Autodesk Fusion 360 part; units mm, degrees
(part 2 of 2)
sketch "Skizze4" plane through (0, 0, 0) normal (0, 1, 0) x (1, 0, 0)
  line L0 (145, 5) -> (150, 5)
  line L1 (150, 5) -> (150, 0)
  line L2 (150, 0) -> (230, 0)
  line L3 (230, 0) -> (230, 5)
  line L4 (230, 5) -> (235, 5)
  line L5 (235, 5) -> (235, 100)
  line L6 (235, 100) -> (145, 100)
  line L7 (145, 100) -> (145, 5)
  line L8 (125, 35) -> (125.0002, 27.0709)
  line L9 (117.9289, 20) -> (137.9289, 0)
  line L10 (145, 0) -> (148.5355, 3.5355) construction
  line L11 (152.0711, 0) -> (172.0709, 19.9998)
  line L12 (165, 35) -> (165, 27.0711)
  line L13 (145, 7.0711) -> (125.0002, 27.0709)
  line L14 (148.5355, -3.5355) -> (180.4271, 28.356) construction
  line L15 (141.4645, 3.5355) -> (172.9289, 35) construction
  line L16 (180, 20) -> (172.0709, 19.9998)
  line L17 (145, 0) -> (141.4645, 3.5355) construction
  line L18 (145, 0) -> (148.5355, -3.5355) construction
  line L19 (141.4645, -3.5355) -> (110, 27.9289) construction
  line L20 (145, -7.0711) -> (164.9998, -27.0709)
  line L21 (141.4645, -3.5355) -> (172.9289, -35) construction
  line L22 (172.0711, -20) -> (152.0711, 0)
  line L23 (110, 35) -> (180, 35) construction
  line L24 (148.5355, -3.5355) -> (117.0711, -35) construction
  line L25 (180, -35) -> (180, -20)
  line L26 (117.9291, -19.9998) -> (110, -19.9998)
  line L27 (180, -35) -> (110, -35) construction
  line L28 (150, 0) -> (150, -5)
  line L29 (180, 20) -> (180, 35)
  line L30 (145, 0) -> (141.4645, -3.5355) construction
  line L31 (180, 35) -> (165, 35)
  line L32 (165, 27.0711) -> (145, 7.0711)
  line L33 (180, 35) -> (110, -35) construction
  line L34 (150, -5) -> (145, -5)
  line L35 (172.0711, -20) -> (180, -20)
  line L36 (164.9998, -35) -> (164.9998, -27.0709)
  line L37 (110, 35) -> (180, -35) construction
  line L38 (110, -35) -> (125, -35)
  line L39 (110, -35) -> (110, 35) construction
  line L40 (164.9998, -35) -> (180, -35)
  line L41 (125, -35) -> (125, -27.0711)
  line L42 (110, -19.9998) -> (110, -35)
  line L43 (110, 35) -> (110, 20)
  line L44 (125, 35) -> (110, 35)
  line L45 (141.4645, 3.5355) -> (110, -27.9289) construction
  line L46 (110, 20) -> (117.9289, 20)
  line L47 (148.5355, 3.5355) -> (180, -27.9289) construction
  line L48 (137.9289, 0) -> (117.9291, -19.9998)
  line L49 (148.5355, 3.5355) -> (117.0711, 35) construction
  line L50 (180, 35) -> (180, -35) construction
  line L51 (125, -27.0711) -> (145, -7.0711)
  line L52 (215, 35) -> (215.0002, 27.0709)
  line L53 (207.9289, 20) -> (227.9289, 0)
  line L54 (235, 0) -> (238.5355, 3.5355) construction
  line L55 (242.0711, 0) -> (262.0709, 19.9998)
  line L56 (255, 35) -> (255, 27.0711)
  line L57 (235, 7.0711) -> (215.0002, 27.0709)
  line L58 (238.5355, -3.5355) -> (270.4271, 28.356) construction
  line L59 (231.4645, 3.5355) -> (262.9289, 35) construction
  line L60 (270, 20) -> (262.0709, 19.9998)
  line L61 (235, 0) -> (231.4645, 3.5355) construction
  line L62 (235, 0) -> (238.5355, -3.5355) construction
  line L63 (231.4645, -3.5355) -> (200, 27.9289) construction
  line L64 (235, -7.0711) -> (254.9998, -27.0709)
  line L65 (231.4645, -3.5355) -> (262.9289, -35) construction
  line L66 (262.0711, -20) -> (242.0711, 0)
  line L67 (200, 35) -> (270, 35) construction
  line L68 (238.5355, -3.5355) -> (207.0711, -35) construction
  line L69 (270, -35) -> (270, -20)
  line L70 (207.9291, -19.9998) -> (200, -19.9998)
  line L71 (270, -35) -> (200, -35) construction
  line L72 (240, 0) -> (240, -5)
  line L73 (270, 20) -> (270, 35)
  line L74 (235, 0) -> (231.4645, -3.5355) construction
  line L75 (270, 35) -> (255, 35)
  line L76 (255, 27.0711) -> (235, 7.0711)
  line L77 (270, 35) -> (200, -35) construction
  line L78 (240, -5) -> (235, -5)
  line L79 (262.0711, -20) -> (270, -20)
  line L80 (254.9998, -35) -> (254.9998, -27.0709)
  line L81 (200, 35) -> (270, -35) construction
  line L82 (200, -35) -> (215, -35)
  line L83 (200, -35) -> (200, 35) construction
  line L84 (254.9998, -35) -> (270, -35)
  line L85 (215, -35) -> (215, -27.0711)
  line L86 (200, -19.9998) -> (200, -35)
  line L87 (200, 35) -> (200, 20)
  line L88 (215, 35) -> (200, 35)
  line L89 (231.4645, 3.5355) -> (200, -27.9289) construction
  line L90 (200, 20) -> (207.9289, 20)
  line L91 (238.5355, 3.5355) -> (270, -27.9289) construction
  line L92 (227.9289, 0) -> (207.9291, -19.9998)
  line L93 (238.5355, 3.5355) -> (207.0711, 35) construction
  line L94 (270, 35) -> (270, -35) construction
  line L95 (215, -27.0711) -> (235, -7.0711)
  line L96 (145, 85) -> (150, 85)
  line L97 (150, 85) -> (150, 95)
  line L98 (150, 95) -> (145, 95)
  line L99 (145, 95) -> (145, 85)
  line L100 (235, 95) -> (230, 95)
  line L101 (230, 95) -> (230, 85)
  line L102 (230, 85) -> (235, 85)
  line L103 (235, 85) -> (235, 95)
  dimension "d109" = 5
  dimension "d110" = 5
  dimension "d111" = 80
  dimension "d112" = 5
  dimension "d113" = 5
  dimension "d115" = 95
  dimension "d116" = 90
  dimension "d117" = 5
  dimension "d118" = 5
  dimension "d119" = 70
  dimension "d120" = 70
  dimension "d121" = 5
  dimension "d122" = 5
  dimension "d123" = 5
  dimension "d124" = 5
  dimension "d125" = 15
  dimension "d126" = 28.284
  dimension "d127" = 28.284
  dimension "d128" = 28.284
  dimension "d129" = 28.284
  dimension "d130" = 5
  dimension "d131" = 5
  dimension "d132" = 70
  dimension "d133" = 70
  dimension "d134" = 5
  dimension "d135" = 5
  dimension "d136" = 5
  dimension "d137" = 5
  dimension "d138" = 15
  dimension "d139" = 28.284
  dimension "d140" = 28.284
  dimension "d141" = 28.284
  dimension "d142" = 28.284
  dimension "d143" = 5
  dimension "d144" = 10
  dimension "d145" = 5
  dimension "d146" = 10
  constraint horizontal L0
  constraint perpendicular L0 L1
  constraint perpendicular L1 L2
  constraint perpendicular L2 L3
  constraint perpendicular L3 L4
  constraint perpendicular L4 L5
  constraint perpendicular L5 L6
  constraint horizontal L23
  constraint vertical L50
  constraint horizontal L27
  constraint vertical L39
  constraint midpoint L10.start L33
  constraint perpendicular L17 L33
  constraint coincident L15.end L23
  constraint perpendicular L15 L37
  constraint coincident L45.end L39
  constraint perpendicular L17 L45
  constraint perpendicular L18 L33
  constraint coincident L24.end L27
  constraint perpendicular L18 L24
  constraint perpendicular L14 L18
  constraint coincident L10.end L33
  constraint coincident L47.end L50
  constraint perpendicular L10 L47
  constraint coincident L49.end L23
  constraint perpendicular L10 L49
  constraint perpendicular L17 L30
  constraint coincident L21.end L27
  constraint perpendicular L21 L33
  constraint coincident L19.end L39
  constraint perpendicular L19 L33
  constraint perpendicular L23 L43
  constraint coincident L9.start L19
  constraint perpendicular L39 L46
  constraint coincident L9.end L19
  constraint coincident L9.end L45
  constraint coincident L26.start L45
  constraint coincident L26.end L39
  constraint perpendicular L26 L39
  constraint coincident L38.end L27
  constraint perpendicular L38 L42
  constraint coincident L41.end L24
  constraint perpendicular L27 L41
  constraint coincident L20.start L21
  constraint coincident L20.start L24
  constraint perpendicular L21 L51
  constraint perpendicular L20 L51
  constraint coincident L36.start L27
  constraint perpendicular L27 L36
  constraint coincident L25.end L50
  constraint perpendicular L25 L40
  constraint coincident L22.start L47
  constraint perpendicular L25 L35
  constraint coincident L11.start L47
  constraint coincident L11.start L14
  constraint perpendicular L14 L22
  constraint perpendicular L11 L47
  constraint coincident L16.start L50
  constraint coincident L12.start L23
  constraint perpendicular L31 L50
  constraint coincident L12.end L15
  constraint perpendicular L12 L23
  constraint coincident L13.start L49
  constraint coincident L13.start L15
  constraint perpendicular L32 L49
  constraint perpendicular L13 L32
  constraint coincident L8.start L23
  constraint horizontal L67
  constraint vertical L94
  constraint horizontal L71
  constraint vertical L83
  constraint midpoint L54.start L77
  constraint perpendicular L61 L77
  constraint coincident L59.end L67
  constraint perpendicular L59 L81
  constraint coincident L89.end L83
  constraint perpendicular L61 L89
  constraint perpendicular L62 L77
  constraint coincident L68.end L71
  constraint perpendicular L62 L68
  constraint perpendicular L58 L62
  constraint coincident L54.end L77
  constraint coincident L91.end L94
  constraint perpendicular L54 L91
  constraint coincident L93.end L67
  constraint perpendicular L54 L93
  constraint perpendicular L61 L74
  constraint coincident L65.end L71
  constraint perpendicular L65 L77
  constraint coincident L63.end L83
  constraint perpendicular L63 L77
  constraint perpendicular L67 L87
  constraint coincident L53.start L63
  constraint perpendicular L83 L90
  constraint coincident L53.end L63
  constraint coincident L53.end L89
  constraint coincident L70.start L89
  constraint coincident L70.end L83
  constraint perpendicular L70 L83
  constraint coincident L82.end L71
  constraint perpendicular L82 L86
  constraint coincident L85.end L68
  constraint perpendicular L71 L85
  constraint coincident L64.start L65
  constraint coincident L64.start L68
  constraint perpendicular L65 L95
  constraint perpendicular L64 L95
  constraint coincident L80.start L71
  constraint perpendicular L71 L80
  constraint coincident L69.end L94
  constraint perpendicular L69 L84
  constraint coincident L66.start L91
  constraint perpendicular L69 L79
  constraint coincident L55.start L91
  constraint coincident L55.start L58
  constraint perpendicular L58 L66
  constraint perpendicular L55 L91
  constraint coincident L60.start L94
  constraint coincident L56.start L67
  constraint perpendicular L75 L94
  constraint coincident L56.end L59
  constraint perpendicular L56 L67
  constraint coincident L57.start L93
  constraint coincident L57.start L59
  constraint perpendicular L76 L93
  constraint perpendicular L57 L76
  constraint coincident L52.start L67
  constraint horizontal L96
  constraint vertical L97
  constraint horizontal L98
  constraint vertical L99
  constraint coincident L7 L96.start
  constraint horizontal L100
  constraint vertical L101
  constraint horizontal L102
  constraint vertical L103
  constraint coincident L5 L100.start
  measures "d109" distance of L0.start L0.end
  measures "d110" distance of L0.end L1.end
  measures "d111" distance of L1.end L2.end
  measures "d112" distance of L2.end L3.end
  measures "d113" distance of L3.end L4.end
  measures "d115" distance of L4.end L5.end
  measures "d116" distance of L5.end L6.end
  measures "d117" distance of L28.end L1.end
  measures "d118" distance of L34.end L28.end
  measures "d119" distance of L23.end L23.start
  measures "d120" distance of L27.end L23.start
  measures "d121" distance of L10.start L15.start
  measures "d122" distance of L10.start L14.start
  measures "d123" distance of L10.end L10.start
  measures "d124" distance of L10.start L19.start
  measures "d125" distance of L23.start L43.end
  measures "d126" distance of L26.start L9.end
  measures "d127" distance of L20.start L20.end
  measures "d128" distance of L11.start L11.end
  measures "d129" distance of L8.end L13.start
  measures "d130" distance of L72.end L72.start
  measures "d131" distance of L78.end L72.end
  measures "d132" distance of L67.end L67.start
  measures "d133" distance of L71.end L67.start
  measures "d134" distance of L54.start L59.start
  measures "d135" distance of L54.start L58.start
  measures "d136" distance of L54.end L54.start
  measures "d137" distance of L54.start L63.start
  measures "d138" distance of L67.start L87.end
  measures "d139" distance of L70.start L53.end
  measures "d140" distance of L64.start L64.end
  measures "d141" distance of L55.start L55.end
  measures "d142" distance of L52.end L57.start
  measures "d143" distance of L96.start L96.end
  measures "d144" distance of L96.start L98.end
  measures "d145" distance of L100.start L100.end
  measures "d146" distance of L100.start L102.end
extrude "Extrusion4" add sketch "Skizze4" along normal blind 10 separate body contours L2 L5 L6 L7 L11 L12 L16 L29 L31 L32 L52 L53 L57 L87 L88 L90 L96 L97 L98 L100 L101 L102 makes body 4
sketch "Skizze5" plane through (0, 0, 0) normal (0, 1, 0) x (1, 0, 0)
  line L0 (145, 5) -> (150, 5)
  line L1 (150, 5) -> (150, 0)
  line L2 (150, 0) -> (230, 0)
  line L3 (230, 0) -> (230, 5)
  line L4 (230, 5) -> (235, 5)
  line L5 (235, 5) -> (235, 45)
  line L6 (235, 45) -> (145, 45)
  line L7 (145, 45) -> (145, 5)
  constraint horizontal L0
  constraint perpendicular L0 L1
  constraint perpendicular L1 L2
  constraint perpendicular L2 L3
  constraint perpendicular L3 L4
  constraint perpendicular L2 L5
  constraint perpendicular L5 L6
  constraint perpendicular L0 L7
extrude "Extrusion5" add sketch "Skizze5" along normal blind 5 bodies 4
sketch "Skizze6" plane through (0, 0, 0) normal (0, 1, 0) x (1, 0, 0)
  line L0 (320, 5) -> (325, 5)
  line L1 (325, 5) -> (325, 0)
  line L2 (325, 0) -> (420, 0)
  line L3 (420, 0) -> (420, 100)
  line L4 (420, 100) -> (320, 100)
  line L5 (320, 100) -> (320, 5)
  line L6 (300, 35) -> (300.0002, 27.0709)
  line L7 (292.9289, 20) -> (312.9289, 0)
  line L8 (320, 0) -> (323.5355, 3.5355) construction
  line L9 (327.0711, 0) -> (347.0709, 19.9998)
  line L10 (340, 35) -> (340, 27.0711)
  line L11 (320, 7.0711) -> (300.0002, 27.0709)
  line L12 (323.5355, -3.5355) -> (355.4271, 28.356) construction
  line L13 (316.4645, 3.5355) -> (347.9289, 35) construction
  line L14 (355, 20) -> (347.0709, 19.9998)
  line L15 (320, 0) -> (316.4645, 3.5355) construction
  line L16 (320, 0) -> (323.5355, -3.5355) construction
  line L17 (316.4645, -3.5355) -> (285, 27.9289) construction
  line L18 (320, -7.0711) -> (339.9998, -27.0709)
  line L19 (316.4645, -3.5355) -> (347.9289, -35) construction
  line L20 (347.0711, -20) -> (327.0711, 0)
  line L21 (285, 35) -> (355, 35) construction
  line L22 (323.5355, -3.5355) -> (292.0711, -35) construction
  line L23 (355, -35) -> (355, -20)
  line L24 (292.9291, -19.9998) -> (285, -19.9998)
  line L25 (355, -35) -> (285, -35) construction
  line L26 (325, 0) -> (325, -5)
  line L27 (355, 20) -> (355, 35)
  line L28 (320, 0) -> (316.4645, -3.5355) construction
  line L29 (355, 35) -> (340, 35)
  line L30 (340, 27.0711) -> (320, 7.0711)
  line L31 (355, 35) -> (285, -35) construction
  line L32 (325, -5) -> (320, -5)
  line L33 (347.0711, -20) -> (355, -20)
  line L34 (339.9998, -35) -> (339.9998, -27.0709)
  line L35 (285, 35) -> (355, -35) construction
  line L36 (285, -35) -> (300, -35)
  line L37 (285, -35) -> (285, 35) construction
  line L38 (339.9998, -35) -> (355, -35)
  line L39 (300, -35) -> (300, -27.0711)
  line L40 (285, -19.9998) -> (285, -35)
  line L41 (285, 35) -> (285, 20)
  line L42 (300, 35) -> (285, 35)
  line L43 (316.4645, 3.5355) -> (285, -27.9289) construction
  line L44 (285, 20) -> (292.9289, 20)
  line L45 (323.5355, 3.5355) -> (355, -27.9289) construction
  line L46 (312.9289, 0) -> (292.9291, -19.9998)
  line L47 (323.5355, 3.5355) -> (292.0711, 35) construction
  line L48 (355, 35) -> (355, -35) construction
  line L49 (300, -27.0711) -> (320, -7.0711)
  line L50 (320, 95) -> (325, 95)
  line L51 (325, 95) -> (325, 85)
  line L52 (325, 85) -> (320, 85)
  line L53 (320, 85) -> (320, 95)
  line L54 (415, 0) -> (405, 0)
  line L55 (405, 0) -> (405, 5)
  line L56 (405, 5) -> (415, 5)
  line L57 (415, 5) -> (415, 0)
  line L58 (415, 95) -> (405, 95)
  line L59 (405, 95) -> (405, 85)
  line L60 (405, 85) -> (415, 85)
  line L61 (415, 85) -> (415, 95)
  dimension "d151" = 95
  dimension "d152" = 100
  dimension "d153" = 100
  dimension "d154" = 5
  dimension "d155" = 5
  dimension "d156" = 70
  dimension "d157" = 70
  dimension "d158" = 5
  dimension "d159" = 5
  dimension "d160" = 5
  dimension "d161" = 5
  dimension "d162" = 15
  dimension "d163" = 28.284
  dimension "d164" = 28.284
  dimension "d165" = 28.284
  dimension "d166" = 28.284
  dimension "d167" = 5
  dimension "d168" = 10
  dimension "d169" = 10
  dimension "d170" = 5
  dimension "d171" = 10
  dimension "d172" = 10
  constraint horizontal L0
  constraint perpendicular L0 L1
  constraint perpendicular L1 L2
  constraint perpendicular L0 L3
  constraint perpendicular L3 L4
  constraint horizontal L21
  constraint vertical L48
  constraint horizontal L25
  constraint vertical L37
  constraint midpoint L8.start L31
  constraint perpendicular L15 L31
  constraint coincident L13.end L21
  constraint perpendicular L13 L35
  constraint coincident L43.end L37
  constraint perpendicular L15 L43
  constraint perpendicular L16 L31
  constraint coincident L22.end L25
  constraint perpendicular L16 L22
  constraint perpendicular L12 L16
  constraint coincident L8.end L31
  constraint coincident L45.end L48
  constraint perpendicular L8 L45
  constraint coincident L47.end L21
  constraint perpendicular L8 L47
  constraint perpendicular L15 L28
  constraint coincident L19.end L25
  constraint perpendicular L19 L31
  constraint coincident L17.end L37
  constraint perpendicular L17 L31
  constraint perpendicular L21 L41
  constraint coincident L7.start L17
  constraint perpendicular L37 L44
  constraint coincident L7.end L17
  constraint coincident L7.end L43
  constraint coincident L24.start L43
  constraint coincident L24.end L37
  constraint perpendicular L24 L37
  constraint coincident L36.end L25
  constraint perpendicular L36 L40
  constraint coincident L39.end L22
  constraint perpendicular L25 L39
  constraint coincident L18.start L19
  constraint coincident L18.start L22
  constraint perpendicular L19 L49
  constraint perpendicular L18 L49
  constraint coincident L34.start L25
  constraint perpendicular L25 L34
  constraint coincident L23.end L48
  constraint perpendicular L23 L38
  constraint coincident L20.start L45
  constraint perpendicular L23 L33
  constraint coincident L9.start L45
  constraint coincident L9.start L12
  constraint perpendicular L12 L20
  constraint perpendicular L9 L45
  constraint coincident L14.start L48
  constraint coincident L10.start L21
  constraint perpendicular L29 L48
  constraint coincident L10.end L13
  constraint perpendicular L10 L21
  constraint coincident L11.start L47
  constraint coincident L11.start L13
  constraint perpendicular L30 L47
  constraint perpendicular L11 L30
  constraint coincident L6.start L21
  constraint horizontal L50
  constraint vertical L51
  constraint horizontal L52
  constraint vertical L53
  constraint coincident L5 L50.start
  constraint horizontal L54
  constraint vertical L55
  constraint horizontal L56
  constraint vertical L57
  constraint coincident L2 L54.start
  constraint horizontal L58
  constraint vertical L59
  constraint horizontal L60
  constraint vertical L61
  measures "d151" distance of L1.end L2.end
  measures "d152" distance of L2.end L3.end
  measures "d153" distance of L3.end L4.end
  measures "d154" distance of L26.end L1.end
  measures "d155" distance of L32.end L26.end
  measures "d156" distance of L21.end L21.start
  measures "d157" distance of L25.end L21.start
  measures "d158" distance of L8.start L13.start
  measures "d159" distance of L8.start L12.start
  measures "d160" distance of L8.end L8.start
  measures "d161" distance of L8.start L17.start
  measures "d162" distance of L21.start L41.end
  measures "d163" distance of L24.start L7.end
  measures "d164" distance of L18.start L18.end
  measures "d165" distance of L9.start L9.end
  measures "d166" distance of L6.end L11.start
  measures "d167" distance of L50.start L50.end
  measures "d168" distance of L50.start L52.end
  measures "d169" distance of L54.start L54.end
  measures "d170" distance of L54.start L56.end
  measures "d171" distance of L58.start L58.end
  measures "d172" distance of L58.start L60.end
extrude "Extrusion6" add sketch "Skizze6" along normal blind 10 separate body contours L2 L3 L4 L5 L9 L10 L14 L27 L29 L30 L50 L51 L52 L55 L56 L57 makes body 5
sketch "Skizze7" plane through (0, 0, 0) normal (0, 1, 0) x (1, 0, 0)
  line L0 (320, 5) -> (325, 5)
  line L1 (325, 5) -> (325, 0)
  line L2 (325, 0) -> (362, 0)
  line L3 (362, 0) -> (362, 40.354)
  line L4 (362, 40.354) -> (320, 40.354)
  line L5 (320, 40.354) -> (320, 5)
  constraint horizontal L0
  constraint perpendicular L0 L1
  constraint perpendicular L1 L2
  constraint perpendicular L2 L3
  constraint perpendicular L1 L4
  constraint perpendicular L0 L5
extrude "Extrusion7" add sketch "Skizze7" along normal blind 5 bodies 5
